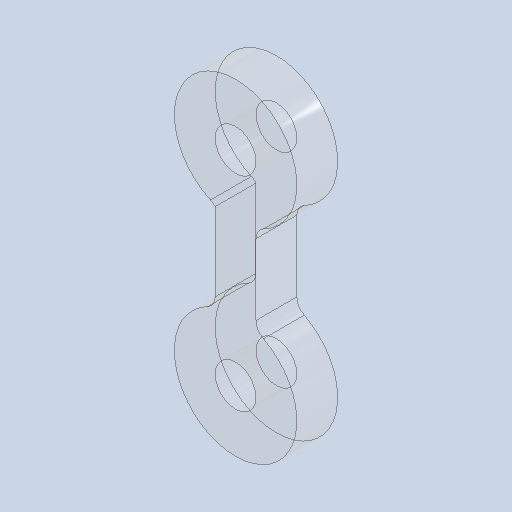
# Autodesk Inventor part: 横wing 押さえ
Saved by Autodesk Inventor 2023 (Build 270158030, 158C)
## iProperties
Created: 2020-05-09
Part Number: 横wing 押さえ
Material: ポリカーボネート、クリア
Document SubType Name: Modeling
Designer: mozar
Density: 1.2 g/cm^3
Appearance: ポリカーボネート - クリア
Author: mozar
Autodesk Inventor part; units mm, degrees
ref_plane "YZ Plane" through (0, 0, 0) normal (1, 0, 0) x (0, 1, 0)
ref_plane "XZ Plane" through (0, 0, 0) normal (0, 1, 0) x (-1, 0, 0)
ref_plane "XY Plane" through (0, 0, 0) normal (0, 0, 1) x (1, 0, 0)
sketch "スケッチ1" plane through (0, 0, 0) normal (0, 0, 1) x (1, 0, 0)
  arc A0 (68.3782, -58.0411) -> (68.9236, -58.9318) centre (69.3782, -58.0411) ccw
  arc A1 (71.3033, -62.1226) -> (68.9236, -58.9318) centre (66.8782, -62.9401) ccw
  arc A2 (71.3033, -62.1226) -> (72.305, -62.9408) centre (72.2867, -61.9409) ccw
  arc A3 (72.3782, -62.9401) -> (72.305, -62.9408) centre (72.3782, -66.9401) ccw
  arc A4 (72.3782, -62.9401) -> (73.3782, -61.9401) centre (72.3782, -61.9401) ccw
  line L0 (73.3782, -61.9401) -> (73.3782, -48.9401)
  arc A5 (73.3782, -48.9401) -> (72.3782, -47.9401) centre (72.3782, -48.9401) ccw
  arc A6 (72.305, -47.9394) -> (72.3782, -47.9401) centre (72.3782, -43.9401) ccw
  arc A7 (72.305, -47.9394) -> (71.3033, -48.7576) centre (72.2867, -48.9393) ccw
  arc A8 (68.9236, -51.9484) -> (71.3033, -48.7576) centre (66.8782, -47.9401) ccw
  arc A9 (68.9236, -51.9484) -> (68.3782, -52.8391) centre (69.3782, -52.8391) ccw
  line L1 (68.3782, -52.8391) -> (68.3782, -58.0411)
  arc A10 (60.3782, -61.9401) -> (61.3782, -62.9401) centre (61.3782, -61.9401) ccw
  arc A11 (61.4514, -62.9408) -> (61.3782, -62.9401) centre (61.3782, -66.9401) ccw
  arc A12 (61.4514, -62.9408) -> (62.4531, -62.1226) centre (61.4697, -61.9409) ccw
  arc A13 (64.8327, -58.9318) -> (62.4531, -62.1226) centre (66.8782, -62.9401) ccw
  arc A14 (64.8327, -58.9318) -> (65.3782, -58.0411) centre (64.3782, -58.0411) ccw
  line L2 (65.3782, -58.0411) -> (65.3782, -52.2984)
  arc A15 (65.3782, -52.2984) -> (65.036, -52.0457) centre (64.6266, -52.9581) ccw
  arc A16 (62.4531, -48.7576) -> (65.036, -52.0457) centre (66.8782, -47.9401) ccw
  arc A17 (62.4531, -48.7576) -> (61.4514, -47.9394) centre (61.4697, -48.9393) ccw
  arc A18 (61.3782, -47.9401) -> (61.4514, -47.9394) centre (61.3782, -43.9401) ccw
  arc A19 (61.3782, -47.9401) -> (60.3782, -48.9401) centre (61.3782, -48.9401) ccw
  line L3 (60.3782, -48.9401) -> (60.3782, -61.9401)
  circle A20 centre (66.8782, -47.9401) radius 1.5
  circle A21 centre (66.8782, -62.9401) radius 1.5
  line L4 (71.3782, -69.9401) -> (62.3782, -69.9401)
  line L5 (62.3782, -69.9401) -> (62.3782, -66.9401)
  arc A22 (62.3782, -66.9401) -> (60.3782, -66.9401) centre (61.3782, -66.9401) ccw
  line L6 (60.3782, -66.9401) -> (57.3782, -66.9401)
  line L7 (57.3782, -66.9401) -> (57.3782, -43.9401)
  line L8 (57.3782, -43.9401) -> (60.3782, -43.9401)
  arc A23 (60.3782, -43.9401) -> (62.3782, -43.9401) centre (61.3782, -43.9401) ccw
  line L9 (62.3782, -43.9401) -> (62.3782, -40.9401)
  line L10 (62.3782, -40.9401) -> (71.3782, -40.9401)
  line L11 (71.3782, -40.9401) -> (71.3782, -43.9401)
  arc A24 (71.3782, -43.9401) -> (73.3782, -43.9401) centre (72.3782, -43.9401) ccw
  line L12 (73.3782, -43.9401) -> (76.3782, -43.9401)
  line L13 (76.3782, -43.9401) -> (76.3782, -66.9401)
  line L14 (76.3782, -66.9401) -> (73.3782, -66.9401)
  arc A25 (73.3782, -66.9401) -> (71.3782, -66.9401) centre (72.3782, -66.9401) ccw
  line L15 (71.3782, -66.9401) -> (71.3782, -69.9401)
  circle A26 centre (66.8782, -47.9401) radius 4.5
  circle A27 centre (66.8782, -62.9401) radius 4.5
  point P0 (0, 0)
  point P1 (0, 0)
  point P2 (62.4531, -48.7576)
  point P3 (62.4531, -62.1226)
  constraints: 48 point on circle, 32 end point, 26 centre point, 10 vertical, 6 horizontal, 2 coincident, 98 other
extrude "押し出し1" add sketch "スケッチ1" against normal blind 3 contours A0 A27 A14 L2 A15 A26 A9 L1 | A1 A27 A13 | A26 A16 A8
